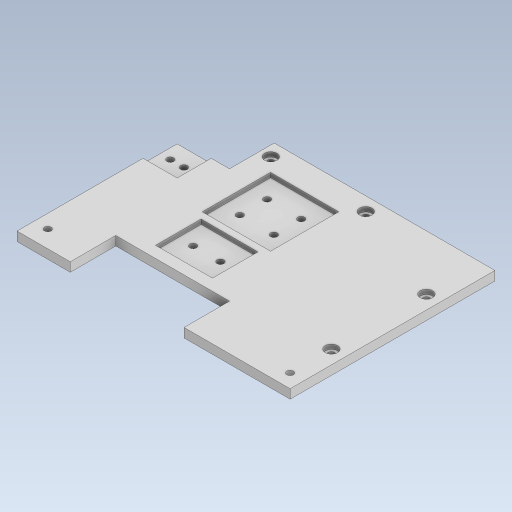
# Autodesk Inventor part: Casis Kiri Atas
Saved by Autodesk Inventor 2023.5 (Build 275446000, 446)
## iProperties
Created: 2025-09-16
Part Number: Casis Kiri Atas
Material: Generic
Document SubType Name: Modeling
Designer: Guntur
Density: 1 g/cm^3
Appearance: Default
Author: Guntur
## iProperties of the stored document Casis Kiri Atas_3DPrint.ipt
Created: 2025-09-19
Part Number: Casis Kiri Atas_3DPrint
Material: Generic
Document SubType Name: Modeling
Designer: Guntur
Density: 1 g/cm^3
Appearance: Default
Author: Guntur
Autodesk Inventor part; units mm, degrees
ref_plane "YZ Plane" through (0, 0, 0) normal (1, 0, 0) x (0, 1, 0)
ref_plane "XZ Plane" through (0, 0, 0) normal (0, 1, 0) x (-1, 0, 0)
ref_plane "XY Plane" through (0, 0, 0) normal (0, 0, 1) x (1, 0, 0)
sketch "Sketch1" plane through (0, 0, 0) normal (0, 1, 0) x (-1, 0, 0)
  line L0 (66.0375, 45) -> (-53.9625, 45)
  line L1 (-53.9625, 45) -> (-53.9625, -45)
  line L2 (66.0375, -45) -> (66.0375, 45)
  line L3 (-53.9625, -45) -> (-5, -45)
  line L4 (5, -45) -> (66.0375, -45)
  line L5 (-53.9625, 0) -> (-53.9625, -5)
  line L6 (-53.9625, -5) -> (-53.9625, 5)
  line L7 (30.1625, 20) -> (5.1625, 20)
  line L8 (5.1625, 20) -> (5.1625, 0)
  line L9 (5.1625, 0) -> (30.1625, 0)
  line L10 (30.1625, 0) -> (30.1625, 20)
  line L11 (32.6625, -3) -> (17.6625, -3)
  line L12 (17.6625, -3) -> (17.6625, -33)
  line L13 (17.6625, -33) -> (32.6625, -33)
  line L14 (32.6625, -33) -> (32.6625, -3)
  circle A0 centre (23.6625, 10) radius 1.5
  circle A1 centre (11.6625, 10) radius 1.5
  circle A2 centre (25.1625, -12) radius 1.5
  circle A3 centre (25.1625, -24) radius 1.5
  line L15 (2.6625, -3) -> (17.6625, -3)
  line L16 (17.6625, -3) -> (17.6625, -33)
  line L17 (17.6625, -33) -> (2.6625, -33)
  line L18 (2.6625, -33) -> (2.6625, -3)
  circle A4 centre (10.1625, -12) radius 1.5
  circle A5 centre (10.1625, -24) radius 1.5
  line L19 (42.6625, 45) -> (-7.3375, 45)
  line L20 (-7.3375, 45) -> (-7.3375, 25)
  line L21 (-7.3375, 25) -> (42.6625, 25)
  line L22 (42.6625, 25) -> (42.6625, 45)
  line L23 (5, -45) -> (-5, -45)
  circle A6 centre (-3.2125, -39) radius 1.5
  circle A7 centre (-3.2125, -39) radius 2.75
  circle A8 centre (38.5375, -39) radius 1.5
  circle A9 centre (38.5375, -39) radius 2.75
  circle A10 centre (-47.9625, 39) radius 1.5
  circle A11 centre (60.0375, 37.5) radius 1.5
  line L24 (66.0375, -45) -> (51.0375, -45)
  line L25 (66.0375, -28) -> (66.0375, -45)
  line L26 (66.0375, -25.35) -> (51.0375, -25.35)
  line L27 (51.0375, -25.35) -> (51.0375, -10.35)
  line L28 (51.0375, -10.35) -> (66.0375, -10.35)
  line L29 (66.0375, -10.35) -> (66.0375, -25.35)
  circle A12 centre (61.5375, -17.85) radius 1.5
  circle A13 centre (61.5375, -17.85) radius 2.5
  circle A14 centre (55.5375, -17.85) radius 1.5
  circle A15 centre (55.5375, -17.85) radius 2.5
  circle A16 centre (-47.9625, 20.875) radius 1.5
  circle A17 centre (-47.9625, -20.875) radius 1.5
  line L30 (-39.6875, 0) -> (-58.7375, 0) construction
  circle A18 centre (-47.9625, 20.875) radius 2.75
  circle A19 centre (-47.9625, -20.875) radius 2.75
  line L31 (17.6625, 0) -> (17.6625, -35.175) construction
  line L32 (51.0375, -25.35) -> (43.0375, -25.35)
  line L33 (43.0375, -25.35) -> (43.0375, -45)
  point P0 (0, 0)
  point P1 (5.1625, 10)
  point P2 (25.1625, -33)
  point P3 (8.375, -33)
  point P4 (-7.3375, 45)
  point P5 (46.0375, -45)
  dimension "d0" = 120
  dimension "d1" = 90
  dimension "d21" = 3
  dimension "d22" = 6.5
  dimension "d23" = 3
  dimension "d24" = 6.5
  dimension "d25" = 3
  dimension "d27" = 3
  dimension "d32" = 5
  dimension "d38" = 3
  dimension "d39" = 5.5
  dimension "d40" = 6
  dimension "d41" = 5.5
  dimension "d42" = 3
  dimension "d43" = 6
  dimension "d44" = 6
  dimension "d45" = 3
  dimension "d46" = 6
  dimension "d59" = 19.65
  dimension "d60" = 3
  dimension "d61" = 5
  dimension "d63" = 7.5
  dimension "d68" = 3
  dimension "d69" = 3
  dimension "d70" = 20.875
  dimension "d71" = 20.875
  dimension "d72" = 5.5
  dimension "d73" = 5.5
  dimension "d74" = 0
  dimension "d75" = 0
  dimension "d76" = 7.5
  dimension "d77" = 7.5
  dimension "d78" = 7.5
  dimension "d79" = 7.5
  dimension "d81" = 8
  constraints: 68 end point, 20 centre point, 11 parallel, 9 horizontal, 6 coincident, 6 perpendicular, 5 point on line, 4 midpoint, 2 vertical
  measures "d0" distance of L2.start L1.end
  measures "d1" distance of L1.end L0.end
  measures "d21" diameter of A0
  measures "d22" distance from line of L10 A0.centre
  measures "d23" diameter of A1
  measures "d24" distance of point (5.163, 10) A1.centre
  measures "d25" diameter of A2
  measures "d27" diameter of A3
  measures "d32" distance between parallel lines of L7 L21
  measures "d38" diameter of A6
  measures "d39" diameter of A7
  measures "d40" distance from line of L3 A6.centre
  measures "d41" diameter of A9
  measures "d42" diameter of A10
  measures "d43" distance from line of L0 A10.centre
  measures "d44" distance from line of L1 A10.centre
  measures "d45" diameter of A11
  measures "d46" distance from line of L2 A11.centre
  measures "d59" distance between parallel lines of L4 L26
  measures "d60" diameter of A12
  measures "d61" diameter of A13
  measures "d63" distance from line of L28 A12.centre
  measures "d68" diameter of A16
  measures "d69" diameter of A17
  measures "d70" distance from line of L30 A16.centre
  measures "d71" distance from line of L30 A17.centre
  measures "d72" diameter of A18
  measures "d73" diameter of A19
  measures "d74" distance between parallel lines of L16 L31
  measures "d75" distance between parallel lines of L31 L12
  measures "d76" distance from line of L18 A4.centre
  measures "d77" distance from line of L12 A2.centre
  measures "d78" distance from line of L12 A3.centre
  measures "d79" distance from line of L18 A5.centre
  measures "d81" distance of L26.end L32.end
extrude "Extrusion3" add sketch "Sketch1" along normal blind 4 contours L2 L28 L27 L32 L33 L4 L23 L3 L1 L0 L20 L21 L22
extrude "Extrusion4" add sketch "Sketch1" along normal blind 2 contours L2 L26 L27 L28 | L10 L9 L8 L7 | L14 L13 L12 L11 | L12 L17 L18 L15 | A7 | A9 | A13 | A15 | A18 | A19
body "Solid2"
